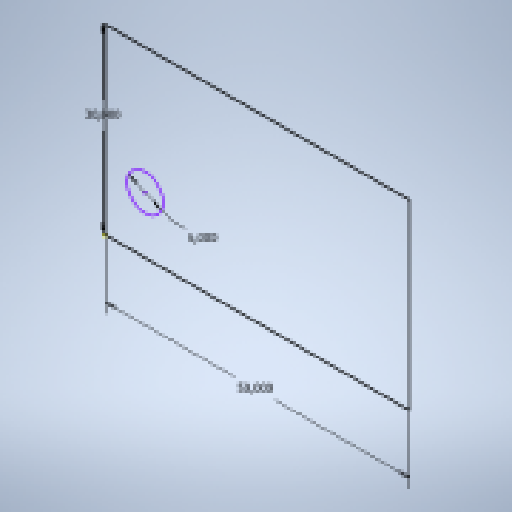
# Autodesk Inventor part: Deska
Saved by Autodesk Inventor 2025.2 (Build 292293000, 293)
## iProperties
Created: 2025-03-23
Part Number: Deska
Material: Wood (Oak)
Document SubType Name: Modeling
Designer: danie
Density: 0.76 g/cm^3
Appearance: White Oak - Natural Medium Gloss
Author: danie
Autodesk Inventor part; units mm, degrees
ref_plane "YZ Plane" through (0, 0, 0) normal (1, 0, 0) x (0, 1, 0)
ref_plane "XZ Plane" through (0, 0, 0) normal (0, 1, 0) x (-1, 0, 0)
ref_plane "XY Plane" through (0, 0, 0) normal (0, 0, 1) x (1, 0, 0)
sketch "Sketch1" plane through (0, 0, 0) normal (0, 0, 1) x (1, 0, 0)
  line L0 (0, 0) -> (1270, 0)
  line L1 (1270, 0) -> (1270, 762)
  line L2 (1270, 762) -> (0, 762)
  line L3 (0, 762) -> (0, 0)
  dimension "d0" = 762
  dimension "d1" = 1270
  constraints: 8 end point, 2 parallel, 1 coincident, 1 horizontal, 1 perpendicular
  measures "d0" distance of L2.end L0.start
  measures "d1" distance of L0.start L0.end
extrude "Extrusion1" add sketch "Sketch1" along normal blind 127
sketch "Sketch2" plane through (0, 0, 127) normal (0, 0, 1) x (1, 0, 0)
  circle A0 centre (381, 381.7881) radius 76.2
  circle A1 centre (634.2119, 127) radius 76.2
  circle A2 centre (889, 380.2119) radius 76.2
  line L0 (0, 0) -> (1270, 0) projected
  line L1 (787.4, 394.1819) -> (990.6, 394.1819)
  line L2 (990.6, 394.1819) -> (990.6, 366.2419)
  line L3 (990.6, 366.2419) -> (787.4, 366.2419)
  line L4 (787.4, 366.2419) -> (787.4, 394.1819)
  line L5 (787.4, 394.1819) -> (990.6, 366.2419) construction
  line L6 (990.6, 394.1819) -> (787.4, 366.2419) construction
  line L7 (279.4, 395.7581) -> (482.6, 395.7581)
  line L8 (482.6, 395.7581) -> (482.6, 367.8181)
  line L9 (482.6, 367.8181) -> (279.4, 367.8181)
  line L10 (279.4, 367.8181) -> (279.4, 395.7581)
  line L11 (279.4, 395.7581) -> (482.6, 367.8181) construction
  line L12 (482.6, 395.7581) -> (279.4, 367.8181) construction
  line L13 (532.6119, 140.97) -> (735.8119, 140.97)
  line L14 (735.8119, 140.97) -> (735.8119, 113.03)
  line L15 (735.8119, 113.03) -> (532.6119, 113.03)
  line L16 (532.6119, 113.03) -> (532.6119, 140.97)
  line L17 (532.6119, 140.97) -> (735.8119, 113.03) construction
  line L18 (735.8119, 140.97) -> (532.6119, 113.03) construction
  point P0 (635, 381)
  point P1 (635, 0)
  point P2 (635, 0)
  point P3 (889, 380.2119)
  point P4 (381, 381.7881)
  point P5 (634.2119, 127)
  point P6 (306.0915, 367.8181)
  point P7 (306.0915, 395.7581)
  point P8 (455.9085, 395.7581)
  point P9 (455.9085, 367.8181)
  point P10 (709.1204, 140.97)
  point P11 (709.1204, 113.03)
  point P12 (559.3034, 113.03)
  point P13 (559.3034, 140.97)
  point P14 (963.9085, 394.1819)
  point P15 (963.9085, 366.2419)
  point P16 (814.0915, 366.2419)
  point P17 (814.0915, 394.1819)
  dimension "d14" = 152.4
  dimension "d17" = 180
  dimension "d19" = 127
  dimension "d20" = 381
  dimension "d23" = 203.2
  dimension "d24" = 27.94
  dimension "d25" = 203.2
  dimension "d26" = 27.94
  dimension "d27" = 203.2
  dimension "d28" = 27.94
  constraints: 36 end point, 8 midpoint, 6 parallel, 3 centre point, 3 coincident, 3 horizontal, 3 perpendicular, 1 vertical alignment, 5 other
  measures "d14" diameter of A0
  measures "d19" distance from line of A1.centre L0
  measures "d20" distance of point (635, 0) point (635, 381)
  measures "d23" distance of L1.start L1.end
  measures "d24" distance of L1.end L2.end
  measures "d25" distance of L7.start L7.end
  measures "d26" distance of L7.end L8.end
  measures "d27" distance of L13.start L13.end
  measures "d28" distance of L13.end L14.end
extrude "Extrusion2" cut sketch "Sketch2" against normal blind 101.6
sketch "Sketch4" plane through (0, 0, 127) normal (0, 0, 1) x (1, 0, 0)
  line L0 (685.0119, 704.85) -> (939.0119, 704.85)
  line L1 (939.0119, 704.85) -> (939.0119, 615.95)
  line L2 (939.0119, 615.95) -> (685.0119, 615.95)
  line L3 (685.0119, 615.95) -> (685.0119, 704.85)
  line L4 (685.0119, 704.85) -> (939.0119, 615.95) construction
  line L5 (939.0119, 704.85) -> (685.0119, 615.95) construction
  line L6 (787.4, 394.1819) -> (814.0915, 394.1819) projected
  arc A0 (963.9085, 394.1819) -> (814.0915, 394.1819) centre (889, 380.2119) ccw projected
  line L7 (963.9085, 394.1819) -> (990.6, 394.1819) projected
  line L8 (990.6, 394.1819) -> (990.6, 366.2419) projected
  line L9 (990.6, 366.2419) -> (963.9085, 366.2419) projected
  arc A1 (814.0915, 366.2419) -> (963.9085, 366.2419) centre (889, 380.2119) ccw projected
  line L10 (814.0915, 366.2419) -> (787.4, 366.2419) projected
  line L11 (787.4, 366.2419) -> (787.4, 394.1819) projected
  line L12 (532.6119, 140.97) -> (559.3034, 140.97) projected
  arc A2 (709.1204, 140.97) -> (559.3034, 140.97) centre (634.2119, 127) ccw projected
  line L13 (709.1204, 140.97) -> (735.8119, 140.97) projected
  line L14 (735.8119, 140.97) -> (735.8119, 113.03) projected
  line L15 (735.8119, 113.03) -> (709.1204, 113.03) projected
  arc A3 (559.3034, 113.03) -> (709.1204, 113.03) centre (634.2119, 127) ccw projected
  line L16 (559.3034, 113.03) -> (532.6119, 113.03) projected
  line L17 (532.6119, 113.03) -> (532.6119, 140.97) projected
  line L18 (482.6, 367.8181) -> (455.9085, 367.8181) projected
  arc A4 (306.0915, 367.8181) -> (455.9085, 367.8181) centre (381, 381.7881) ccw projected
  line L19 (306.0915, 367.8181) -> (279.4, 367.8181) projected
  line L20 (279.4, 367.8181) -> (279.4, 395.7581) projected
  line L21 (279.4, 395.7581) -> (306.0915, 395.7581) projected
  arc A5 (455.9085, 395.7581) -> (306.0915, 395.7581) centre (381, 381.7881) ccw projected
  line L22 (455.9085, 395.7581) -> (482.6, 395.7581) projected
  line L23 (482.6, 395.7581) -> (482.6, 367.8181) projected
  line L24 (1270, 0) -> (1270, 762) projected
  line L25 (1270, 762) -> (0, 762) projected
  line L26 (0, 762) -> (0, 0) projected
  line L27 (0, 0) -> (1270, 0) projected
  line L28 (532.6119, 140.97) -> (532.6119, 113.03) projected
  line L29 (532.6119, 113.03) -> (559.3034, 113.03) projected
  arc A6 (559.3034, 113.03) -> (709.1204, 113.03) centre (634.2119, 127) ccw projected
  line L30 (709.1204, 113.03) -> (735.8119, 113.03) projected
  line L31 (735.8119, 113.03) -> (735.8119, 140.97) projected
  line L32 (735.8119, 140.97) -> (709.1204, 140.97) projected
  arc A7 (709.1204, 140.97) -> (559.3034, 140.97) centre (634.2119, 127) ccw projected
  line L33 (559.3034, 140.97) -> (532.6119, 140.97) projected
  line L34 (329.4119, 704.85) -> (583.4119, 704.85)
  line L35 (583.4119, 704.85) -> (583.4119, 615.95)
  line L36 (583.4119, 615.95) -> (329.4119, 615.95)
  line L37 (329.4119, 615.95) -> (329.4119, 704.85)
  line L38 (329.4119, 704.85) -> (583.4119, 615.95) construction
  line L39 (583.4119, 704.85) -> (329.4119, 615.95) construction
  line L40 (583.4119, 330.9881) -> (685.0119, 330.9881)
  line L41 (685.0119, 330.9881) -> (685.0119, 432.5881)
  line L42 (685.0119, 432.5881) -> (583.4119, 432.5881)
  line L43 (583.4119, 432.5881) -> (583.4119, 330.9881)
  line L44 (583.4119, 330.9881) -> (685.0119, 432.5881) construction
  line L45 (685.0119, 330.9881) -> (583.4119, 432.5881) construction
  point P0 (812.0119, 660.4)
  point P1 (634.2119, 653.1699)
  point P2 (456.4119, 660.4)
  point P3 (634.2119, 381.7881)
  dimension "d29" = 254
  dimension "d30" = 88.9
  dimension "d31" = 177.8
  dimension "d32" = 101.6
  dimension "d33" = 254
  dimension "d34" = 88.9
  dimension "d35" = 177.8
  dimension "d36" = 101.6
  dimension "d37" = 101.6
  dimension "d38" = 101.6
  constraints: 36 end point, 6 midpoint, 6 parallel, 3 horizontal, 3 perpendicular, 2 vertical alignment, 1 horizontal alignment
  measures "d29" distance of L0.start L0.end
  measures "d30" distance of L0.end L1.end
  measures "d31" horizontal distance of point (812.012, 660.4) point (634.212, 653.17)
  measures "d32" distance from line of L25 point (812.012, 660.4)
  measures "d33" distance of L37.end L39.start
  measures "d34" distance of L39.start L36.start
  measures "d35" horizontal distance of point (634.212, 653.17) point (456.412, 660.4)
  measures "d36" distance from line of L25 point (456.412, 660.4)
  measures "d37" distance of L41.end L42.end
  measures "d38" distance of L40.end L41.end
extrude "Extrusion3" add sketch "Sketch4" along normal blind 25.4 contours L0 L1 L2 L3 | L34 L35 L36 L37 | L43 L42 L41 L40
body "Solid1"
